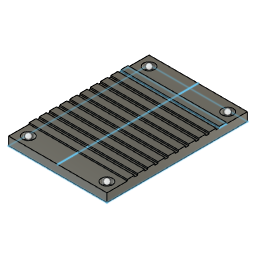
Scales parallel lines (Autodesk Fusion 360 design; units mm, degrees)
Autodesk Fusion 360 part; units mm, degrees
sketch "sketch 584" plane through (-0.0064, 66.4929, 16.5) normal (0, 0, 1) x (1, 0, 0)
  line L0 (35, -50) -> (35, 50)
  line L1 (35, 50) -> (-35, 50)
  line L2 (-35, 50) -> (-35, -50)
  line L3 (-35, -50) -> (35, -50)
extrude "Extrude1" add sketch "sketch 584" along normal blind 6
sketch "sketch 573" plane through (-0.0064, 66.4929, 22.5) normal (0, 0, 1) x (1, 0, 0)
  line L0 (0, 50) -> (0, -50)
  line L1 (0, 50) -> (0, -50)
  line L2 (35, 30) -> (-35, 30)
  line L3 (35, 35) -> (35, 30)
  line L4 (-35, 35) -> (35, 35)
  line L5 (-35, 30) -> (-35, 35)
extrude "Extrude2" add sketch "sketch 573" along normal blind 1
pattern_path "PathPattern1" count 10 spacing 7.2706 from (-0.0064, 98.9929, 22.5) path "sketch 573" along L0 of "Extrude2"
hole "Hole1" at (27.9936, 23.4929, 22.5) at (-28.0064, 23.4929, 22.5) at (-28.0064, 109.4929, 22.5) at (27.9936, 109.4929, 22.5) direction (0, 0, -1) diameter 5 depth 9 tip angle 118 counterbore diameter 8 counterbore depth 4.5
